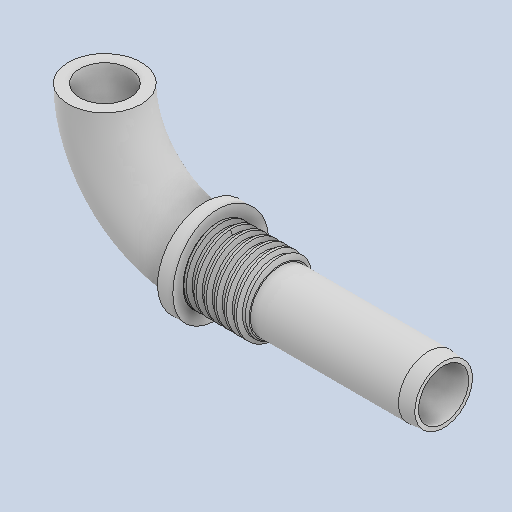
# Autodesk Inventor part: pipe_angle
Saved by Autodesk Inventor 2025 (Build 290162000, 162)
## iProperties
Created: 2026-04-07
Part Number: pipe_angle
Material: Generic
Document SubType Name: Modeling
Designer: Luca
Density: 1 g/cm^3
Appearance: Default
Author: Luca
Autodesk Inventor part; units mm, degrees
ref_plane "YZ Plane" through (0, 0, 0) normal (1, 0, 0) x (0, 1, 0)
ref_plane "XZ Plane" through (0, 0, 0) normal (0, 1, 0) x (-1, 0, 0)
ref_plane "XY Plane" through (0, 0, 0) normal (0, 0, 1) x (1, 0, 0)
derived "sk_reservoir.ipt"
sketch "pipe_out" plane through (-77.5, 0, 0) normal (1, 0, 0) x (0, 1, 0)
  line L0 (-132, 0) -> (302, 0) construction
  circle A0 centre (-10, 0) radius 7.5
  line L1 (0, 153.4424) -> (0, -148.4939) construction
  circle A1 centre (-10, 0) radius 7.25
  circle A2 centre (-10, 0) radius 5
  circle A3 centre (-10, 0) radius 9.5
  circle A4 centre (-10, 0) radius 6
  circle A5 centre (-10, 0) radius 6.25
  circle A6 centre (-10, 0) radius 9.75
  point P0 (0, 0)
  point P1 (-2.5, 0)
  point P2 (-2.75, 0)
sketch "walls" plane through (0, -70, 0) normal (0, 1, 0) x (-1, 0, 0)
  circle A0 centre (0, 0) radius 80
  line L0 (38, -69.4029) -> (38, 38)
  line L1 (38, 38) -> (-69.4029, 38)
  line L2 (35, -68.5857) -> (35, 35)
  line L3 (35, 35) -> (-68.5857, 35)
  arc A1 (-68.5857, 35) -> (35, -68.5857) centre (0, 0) ccw
  arc A2 (38.25, -67.9775) -> (-67.9775, 38.25) centre (0, 0) ccw
  line L4 (80, 0) -> (-80, 0) construction
  line L5 (0, -80) -> (0, 80) construction
  arc A3 (57.0831, 54.4315) -> (54.4315, 57.0831) centre (0, 0) ccw
  line L6 (57.0831, 54.4315) -> (57.8788, 55.2272)
  arc A4 (57.0871, 54.7889) -> (54.427, 57.4322) centre (0, 0) ccw
  line L7 (57.706, 55.4078) -> (57.0871, 54.7889)
  line L8 (38.25, -68.9797) -> (38.25, 38.25)
  line L9 (38.25, 38.25) -> (-68.9797, 38.25)
  line L10 (0, 0) -> (56.5685, 56.5685) construction
  line L11 (54.4315, 57.0831) -> (35.5983, 38.25)
  line L12 (54.427, 57.4322) -> (35.2448, 38.25)
  arc A5 (-67.18, 41.3294) -> (-68.9797, 38.25) centre (0, 0) ccw
  arc A6 (-67.524, 41.2465) -> (-69.4029, 38) centre (0, 0) ccw
  line L13 (-67.18, 41.3294) -> (-68.14, 41.9158)
  line L14 (-67.524, 41.2465) -> (-68.2707, 41.7027)
  arc A7 (38, -69.4029) -> (41.2465, -67.524) centre (0, 0) ccw
  line L15 (41.2465, -67.524) -> (41.7027, -68.2707)
  arc A8 (38.25, -68.9797) -> (41.3294, -67.18) centre (0, 0) ccw
  line L16 (41.3294, -67.18) -> (41.9158, -68.14)
  point P0 (35.8974, -71.4939)
  point P1 (53.8126, 56.4642)
  point P2 (-67.9775, 38.25)
extrude "Extrusion5" add sketch "pipe_out" against normal blind 5 contours A0 | A1 | A3 | A4 | A5
extrude "Extrusion6" cut sketch "walls" along normal through all contours A0 L16 A8 L8 A2 L11 A3 L6 | L6 A3 L11 A2 L12 A4 L7 A0 | A0 L15 A7 L0 L1 A6 L14 L13 A5 L9 L8 A8 L16 | L7 A4 L12 A2 L9 A5 L13 A0 | A0 L14 A6 L1 L0 A7 L15 | L11 L9 L12 A2 | A2 L8 L9 L11 | L12 L9 A2 | A1 L3 L2
sketch "Sketch22" plane through (0, 0, 0) normal (0, 0, 1) x (1, 0, 0)
  line L0 (-77.5, -10) -> (-82.5, -10) projected
  arc A0 (-102.5, 10) -> (-82.5, -10) centre (-82.5, 10) ccw projected
  line L1 (-77.5, -10) -> (-67.5, -10) projected
  line L2 (-77.5, -2.75) -> (-76, -2.75) projected
  line L3 (-76.433, -3.5) -> (-77.067, -3.5) projected
  line L4 (-76.25, -2.75) -> (-76.5387, -3.25) projected
  line L5 (-76.5387, -3.25) -> (-76.9613, -3.25) projected
  line L6 (-76.9613, -3.25) -> (-77.25, -2.75) projected
  line L7 (-76.75, -2.75) -> (-76.75, -3.5) construction
  line L8 (-76, -2.75) -> (-76.433, -3.5) projected
  line L9 (-77.5, -2.75) -> (-77.067, -3.5) projected
  point P0 (0, 0)
  point P1 (-77.5, -2.5)
sweep "Sweep2" add profiles "pipe_out" path "Sketch22" path curves L1 L0 A0 contours A1 | A4 | A5
chamfer "Chamfer2" distance 1 distance2 1 1 edges at (-67.5, -17.25, 0) measured on face at (-67.5, -16.75, 0)
coil "Coil1" sketch "Sketch22" operation cut axis through (-77.5, -10, 0) along (1, 0, 0) pitch 2 turns 5 hand right
coil "Coil2" sketch "Sketch22" operation cut axis through (-77.5, -10, 0) along (-1, 0, 0) pitch 2 turns 2 hand right
extrude "Extrusion8" add sketch "pipe_out" along normal blind 42.5 contours A4
chamfer "Chamfer3" distance 0.25 distance2 3 1 edges at (-35, -16, 0) measured on face at (-35, -15.5, 0)
body "Solid3"
body "Solid4"
